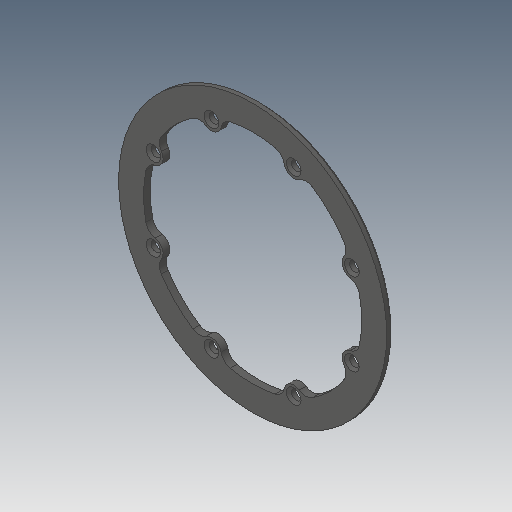
# Autodesk Inventor part: UPPER_TIMING_PULLEY_COVER_OUTER
Saved by Autodesk Inventor 2019.4 (Build 234330000, 330)
## iProperties
Created: 2019-11-12
Part Number: UPPER_TIMING_PULLEY_COVER_OUTER
Material: 一般
Document SubType Name: Modeling
Designer: y6tada
Density: 1 g/cm^3
Appearance: Black 100
Mass: 0.434585 g
Surface Area: 11.3068 cm^2
Volume: 0.434585 cm^3
Author: y6tada
Autodesk Inventor part; units mm, degrees
ref_plane "YZ Plane" through (0, 0, 0) normal (1, 0, 0) x (0, 1, 0)
ref_plane "XZ Plane" through (0, 0, 0) normal (0, 1, 0) x (-1, 0, 0)
ref_plane "XY Plane" through (0, 0, 0) normal (0, 0, 1) x (1, 0, 0)
sketch "スケッチ1" plane through (0, 0, 0) normal (0, 0, 1) x (1, 0, 0)
  circle A0 centre (0, 0) radius 19.97
  arc A1 (-1.2242, 18.6799) -> (-1.7131, 18.6415) centre (0, 0) ccw construction
  circle A2 centre (-6.1229, 14.7821) radius 0.5915 construction
  circle A3 centre (0, 0) radius 16.25
  dimension "d2" = 1.25
  dimension "d6" = 32.5
  constraints: 2 centre point, 2 coincident
  measures "d2" radial gap between concentric circles of A0 A1
  measures "d6" diameter of A3
extrude "押し出し1" add sketch "スケッチ1" along normal blind 1
sketch "スケッチ2" plane through (0, 0, 0) normal (0, 0, 1) x (1, 0, 0)
  circle A0 centre (-6.1229, 14.7821) radius 0.5915 construction
  circle A1 centre (-6.1229, 14.7821) radius 1.45
  point P0 (0, 0)
  dimension "d7" = 2.9
  constraints: 2 coincident, 1 centre point
  measures "d7" diameter of A1
extrude "押し出し2" add sketch "スケッチ2" along normal blind 1
fillet "フィレット1" radius 1.75 2 edges at (-7.5227, 14.4039, 0.5) (-4.8657, 15.5044, 0.5)
sketch "スケッチ3" plane through (0, 0, 1) normal (0, 0, 1) x (1, 0, 0)
  arc A0 (-6.9412, 13.585) -> (-4.6979, 14.5142) centre (-6.1229, 14.7821) ccw construction
  point P0 (0, 0)
  constraints: 1 coincident
hole "穴2" at (-6.1229, 14.7821, 1) direction (0, 0, -1) diameter 1.45 end through all countersink diameter 2.2 countersink angle 90
pattern_circular "円形状パターン1" count 8 over 360 about axis through (0, 0, -10) along (0, 0, 1) of "フィレット1", "押し出し2", "穴2"
chamfer "面取り1" distance 0.4 angle 45 1 edges at (-19.97, 0, 0)
